kindle-calendar-v0.2 (Autodesk Fusion 360 design; units mm, degrees)
part number: 2026-08-25-10-04-39-781
part number: 2026-08-25-10-04-40-282
part number: 2026-08-25-10-04-41-157
part number: 2026-08-25-10-04-41-332
part number: 2026-08-25-10-04-41-515
part number: 2026-08-25-10-04-41-590
part number: 2026-08-25-10-04-41-668
Autodesk Fusion 360 part; units mm, degrees
sketch "Outer biomorphic silhouette" plane through (0, 0, 0) normal (0, 0, 1) x (1, 0, 0) in component "01 Asymmetric Front Shell"
  spline S0 degree 5 poles (-110, 58) (-109.8536, 58.1992) (-109.5513, 58.5949) (-109.0687, 59.1811) (-108.3683, 59.9478) (-107.4137, 60.8802) (-106.4012, 61.7844) (-105.3501, 62.6585) (-104.2698, 63.5023) (-103.1612, 64.3169) (-102.0207, 65.104) (-100.843, 65.8656) (-99.6254, 66.6035) (-98.369, 67.3186) (-97.0773, 68.0113) (-95.7548, 68.682) (-94.406, 69.3309) (-93.0336, 69.9586) (-91.6389, 70.5656) (-90.2223, 71.1528) (-88.7835, 71.7209) (-87.3225, 72.2707) (-85.8396, 72.8028) (-84.3357, 73.3177) (-82.8123, 73.8158) (-81.2704, 74.2975) (-79.7114, 74.7631) (-78.1363, 75.213) (-76.5457, 75.6475) (-74.9401, 76.0671) (-73.3198, 76.472) (-71.6854, 76.8628) (-70.0371, 77.2395) (-68.3753, 77.6027) (-66.7008, 77.9525) (-65.014, 78.2891) (-63.3154, 78.6129) (-61.6055, 78.9239) (-59.8849, 79.2225) (-58.154, 79.5088) (-56.413, 79.7831) (-54.6623, 80.0454) (-52.9022, 80.2961) (-51.1331, 80.5352) (-49.3552, 80.7629) (-47.569, 80.9795) (-45.7747, 81.1849) (-43.9727, 81.3794) (-42.1632, 81.5631) (-40.3466, 81.7361) (-38.5232, 81.8984) (-36.6932, 82.0503) (-34.8569, 82.1918) (-33.0145, 82.323) (-31.1664, 82.4441) (-29.3127, 82.555) (-27.4537, 82.6559) (-25.5896, 82.7469) (-23.7207, 82.828) (-21.8472, 82.8993) (-19.9693, 82.9608) (-18.0873, 83.0127) (-16.2014, 83.055) (-14.3119, 83.0877) (-12.4188, 83.1108) (-10.5225, 83.1245) (-8.6232, 83.1287) (-6.721, 83.1236) (-4.8162, 83.109) (-2.9089, 83.0852) (-0.9993, 83.052) (0.9123, 83.0096) (2.8257, 82.9579) (4.7408, 82.897) (6.6574, 82.8269) (8.5752, 82.7476) (10.4939, 82.659) (12.4135, 82.5612) (14.3337, 82.4542) (16.2544, 82.338) (18.1754, 82.2127) (20.0965, 82.0781) (22.0176, 81.9344) (23.9386, 81.7816) (25.8592, 81.6196) (27.7793, 81.4484) (29.6985, 81.268) (31.6165, 81.0782) (33.5331, 80.879) (35.4479, 80.6704) (37.3608, 80.4523) (39.2716, 80.2247) (41.1804, 79.9878) (43.0872, 79.7414) (44.9921, 79.4858) (46.8951, 79.221) (48.796, 78.9469) (50.6944, 78.6634) (52.5898, 78.3703) (54.4812, 78.0673) (56.3678, 77.754) (58.2491, 77.4301) (60.1245, 77.0957) (61.9943, 76.7506) (63.8591, 76.3953) (65.7201, 76.0303) (67.5784, 75.656) (69.4351, 75.273) (71.2902, 74.8814) (73.143, 74.4807) (74.991, 74.07) (76.8309, 73.6477) (78.659, 73.2124) (80.4724, 72.7628) (82.2696, 72.2982) (84.0519, 71.8192) (85.8237, 71.3278) (87.5923, 70.827) (89.3653, 70.3201) (91.1485, 69.8097) (92.944, 69.2966) (94.7479, 68.7792) (96.5478, 68.252) (98.3255, 67.7073) (100.0622, 67.1368) (101.7442, 66.5346) (103.3671, 65.899) (104.9414, 65.2342) (106.4984, 64.5538) (108.0806, 63.8762) (109.7297, 63.2194) (111.4739, 62.5956) (113.3164, 62.006) (115.2224, 61.4358) (117.1099, 60.8495) (118.8737, 60.2015) (120.4065, 59.4454) (121.6228, 58.5441) (122.4786, 57.4779) (122.9997, 56.2572) (123.2769, 54.9205) (123.4272, 53.5172) (123.5655, 52.0965) (123.7693, 50.6918) (124.054, 49.3103) (124.3966, 47.9433) (124.7539, 46.5733) (125.0817, 45.1826) (125.3572, 43.762) (125.5811, 42.3127) (125.7671, 40.8409) (125.9346, 39.3553) (126.101, 37.8636) (126.2728, 36.3692) (126.4483, 34.8719) (126.621, 33.3695) (126.7829, 31.8589) (126.9273, 30.3379) (127.0523, 28.8062) (127.1592, 27.2646) (127.2508, 25.7149) (127.3308, 24.159) (127.4019, 22.5985) (127.465, 21.034) (127.5196, 19.4659) (127.5644, 17.894) (127.5979, 16.3181) (127.619, 14.738) (127.6273, 13.154) (127.6229, 11.5666) (127.6064, 9.9763) (127.5784, 8.3839) (127.5393, 6.7898) (127.4893, 5.1945) (127.4283, 3.5985) (127.3559, 2.002) (127.2718, 0.4052) (127.1757, -1.1915) (127.0675, -2.788) (126.947, -4.3838) (126.8142, -5.9786) (126.6692, -7.572) (126.5119, -9.1635) (126.3422, -10.7526) (126.16, -12.339) (125.9651, -13.9221) (125.7573, -15.5016) (125.5363, -17.077) (125.302, -18.6481) (125.0543, -20.2147) (124.7929, -21.7765) (124.5177, -23.3334) (124.2285, -24.8846) (123.925, -26.4296) (123.607, -27.9673) (123.2741, -29.4968) (122.926, -31.0172) (122.5624, -32.5281) (122.1832, -34.0297) (121.7881, -35.5227) (121.377, -37.0074) (120.9497, -38.4841) (120.5056, -39.9519) (120.0444, -41.4085) (119.5652, -42.8504) (119.0673, -44.2743) (118.5502, -45.678) (118.0136, -47.0616) (117.4574, -48.4288) (116.882, -49.7855) (116.2877, -51.1365) (115.6741, -52.4832) (115.0403, -53.8207) (114.3843, -55.1352) (113.7035, -56.4096) (112.996, -57.6312) (112.2611, -58.797) (111.5002, -59.9229) (110.717, -61.0429) (109.915, -62.1908) (109.0958, -63.3842) (108.2575, -64.6092) (107.3916, -65.8006) (106.4871, -66.8662) (105.5344, -67.7206) (104.5298, -68.3118) (103.4799, -68.6609) (102.4017, -68.8585) (101.3139, -69.0113) (100.2312, -69.2048) (99.157, -69.4545) (98.087, -69.7325) (97.0134, -69.9954) (95.9293, -70.2157) (94.8311, -70.3967) (93.7186, -70.5537) (92.5947, -70.7053) (91.4659, -70.8577) (90.3388, -71.0076) (89.2161, -71.1477) (88.0919, -71.2722) (86.9489, -71.3805) (85.771, -71.4751) (84.5521, -71.5599) (83.3097, -71.6374) (82.084, -71.7082) (80.9096, -71.7718) (79.7971, -71.8272) (78.7032, -71.8739) (77.537, -71.9118) (76.1974, -71.9414) (74.6001, -71.9637) (72.715, -71.9795) (70.5721, -71.9899) (68.2401, -71.9961) (65.812, -71.9993) (63.389, -72.0003) (61.0632, -72.0003) (58.9037, -71.9998) (56.9362, -71.9993) (55.142, -71.9992) (53.4753, -71.9993) (51.8752, -71.9996) (50.2802, -72) (48.6412, -72.0003) (46.9367, -72.0004) (45.1685, -72.0004) (43.3535, -72.0003) (41.5165, -72.0001) (39.6833, -72) (37.8724, -71.9999) (36.0898, -71.9998) (34.3326, -71.9998) (32.5923, -71.9999) (30.8576, -72) (29.1182, -72) (27.3678, -72.0001) (25.6053, -72.0001) (23.8329, -72.0001) (22.0548, -72) (20.276, -72) (18.5004, -72) (16.7299, -72) (14.9644, -72) (13.2026, -72) (11.4423, -72) (9.6817, -72) (7.9191, -72) (6.1544, -72) (4.3877, -72) (2.62, -72) (0.8522, -72) (-0.915, -72) (-2.6811, -72) (-4.4465, -72) (-6.2115, -72) (-7.9767, -72) (-9.7427, -72) (-11.5095, -72) (-13.2767, -72) (-15.0438, -72.0001) (-16.8099, -72.0001) (-18.5744, -72) (-20.3372, -72) (-22.0988, -71.9999) (-23.8606, -71.9999) (-25.6242, -71.9998) (-27.391, -71.9999) (-29.1619, -71.9999) (-30.9365, -72.0001) (-32.7126, -72.0002) (-34.4867, -72.0003) (-36.2552, -72.0004) (-38.015, -72.0003) (-39.7654, -72.0001) (-41.5084, -71.9997) (-43.2504, -71.9994) (-45, -71.9992) (-46.7655, -71.9992) (-48.5525, -71.9995) (-50.3617, -72.0001) (-52.1857, -72.0009) (-54.0082, -72.0019) (-55.8082, -72.0025) (-57.5645, -72.0026) (-59.2593, -72.0015) (-60.8822, -71.9988) (-62.4358, -71.9938) (-63.9338, -71.986) (-65.3961, -71.9748) (-66.8432, -71.9595) (-68.2915, -71.9398) (-69.7476, -71.9154) (-71.2093, -71.886) (-72.6694, -71.8516) (-74.1192, -71.8122) (-75.5518, -71.768) (-76.9654, -71.7192) (-78.3613, -71.6659) (-79.743, -71.6083) (-81.1137, -71.5459) (-82.4753, -71.4782) (-83.8275, -71.4043) (-85.1688, -71.3233) (-86.4975, -71.2349) (-87.8119, -71.1397) (-89.1112, -71.0391) (-90.3952, -70.9349) (-91.6641, -70.8275) (-92.9185, -70.7157) (-94.1589, -70.5951) (-95.3857, -70.4612) (-96.5986, -70.3116) (-97.7964, -70.1486) (-98.9764, -69.9814) (-100.1362, -69.8199) (-101.2743, -69.6687) (-102.3923, -69.5197) (-103.4947, -69.3489) (-104.5859, -69.1268) (-105.6673, -68.8256) (-106.733, -68.43) (-107.7721, -67.9375) (-108.7723, -67.3527) (-109.7243, -66.6839) (-110.6256, -65.9382) (-111.4785, -65.122) (-112.2874, -64.241) (-113.0566, -63.3006) (-113.7878, -62.3059) (-114.4821, -61.2616) (-115.1394, -60.1723) (-115.7605, -59.0417) (-116.3468, -57.8734) (-116.9003, -56.6703) (-117.4232, -55.4349) (-117.9176, -54.1697) (-118.3848, -52.8767) (-118.8262, -51.5579) (-119.2426, -50.2152) (-119.6348, -48.8502) (-120.0038, -47.4645) (-120.3505, -46.0593) (-120.6757, -44.636) (-120.9805, -43.1957) (-121.2656, -41.7396) (-121.5317, -40.2685) (-121.7796, -38.7835) (-122.0098, -37.2855) (-122.2227, -35.7753) (-122.4188, -34.2537) (-122.5987, -32.7216) (-122.7628, -31.1795) (-122.9115, -29.6283) (-123.0452, -28.0686) (-123.1643, -26.501) (-123.2691, -24.9262) (-123.3601, -23.3447) (-123.4374, -21.7571) (-123.5013, -20.164) (-123.5522, -18.5659) (-123.5901, -16.9633) (-123.6155, -15.3568) (-123.6284, -13.7469) (-123.629, -12.1341) (-123.6176, -10.5188) (-123.5944, -8.9016) (-123.5595, -7.2829) (-123.513, -5.6633) (-123.4552, -4.0431) (-123.386, -2.4228) (-123.3057, -0.803) (-123.2143, 0.8159) (-123.1118, 2.4336) (-122.9983, 4.0494) (-122.874, 5.663) (-122.7388, 7.2738) (-122.593, 8.8813) (-122.4365, 10.4852) (-122.2695, 12.0848) (-122.0919, 13.6796) (-121.9038, 15.2692) (-121.705, 16.8531) (-121.4953, 18.4308) (-121.2746, 20.0019) (-121.0429, 21.5656) (-120.8002, 23.1215) (-120.5467, 24.6688) (-120.2827, 26.2069) (-120.0083, 27.7351) (-119.7235, 29.2526) (-119.4279, 30.7589) (-119.1205, 32.2534) (-118.8005, 33.7357) (-118.4671, 35.2052) (-118.12, 36.6609) (-117.7599, 38.1017) (-117.3881, 39.5263) (-117.0062, 40.9331) (-116.6149, 42.3206) (-116.2133, 43.6879) (-115.7983, 45.0346) (-115.3649, 46.3605) (-114.9088, 47.6654) (-114.4282, 48.948) (-113.9259, 50.2053) (-113.4109, 51.4327) (-112.8926, 52.6248) (-112.3754, 53.7773) (-111.8541, 54.8885) (-111.3076, 55.9605) (-110.8269, 56.7905) (-110.4297, 57.3999) (-110.1464, 57.8008) (-110, 58) knots 0 0 0 0 0 0 0.00222222 0.00444444 0.00666667 0.00888889 0.01111111 0.01333333 0.01555556 0.01777778 0.02 0.02222222 0.02444444 0.02666667 0.02888889 0.03111111 0.03333333 0.03555556 0.03777778 0.04 0.04222222 0.04444444 0.04666667 0.04888889 0.05111111 0.05333333 0.05555556 0.05777778 0.06 0.06222222 0.06444444 0.06666667 0.06888889 0.07111111 0.07333333 0.07555556 0.07777778 0.08 0.08222222 0.08444444 0.08666667 0.08888889 0.09111111 0.09333333 0.09555556 0.09777778 0.1 0.10222222 0.10444444 0.10666667 0.10888889 0.11111111 0.11333333 0.11555556 0.11777778 0.12 0.12222222 0.12444444 0.12666667 0.12888889 0.13111111 0.13333333 0.13555556 0.13777778 0.14 0.14222222 0.14444444 0.14666667 0.14888889 0.15111111 0.15333333 0.15555556 0.15777778 0.16 0.16222222 0.16444444 0.16666667 0.16888889 0.17111111 0.17333333 0.17555556 0.17777778 0.18 0.18222222 0.18444444 0.18666667 0.18888889 0.19111111 0.19333333 0.19555556 0.19777778 0.2 0.20222222 0.20444444 0.20666667 0.20888889 0.21111111 0.21333333 0.21555556 0.21777778 0.22 0.22222222 0.22444444 0.22666667 0.22888889 0.23111111 0.23333333 0.23555556 0.23777778 0.24 0.24222222 0.24444444 0.24666667 0.24888889 0.25111111 0.25333333 0.25555556 0.25777778 0.26 0.26222222 0.26444444 0.26666667 0.26888889 0.27111111 0.27333333 0.27555556 0.27777778 0.28 0.28222222 0.28444444 0.28666667 0.28888889 0.29111111 0.29333333 0.29555556 0.29777778 0.3 0.30222222 0.30444444 0.30666667 0.30888889 0.31111111 0.31333333 0.31555556 0.31777778 0.32 0.32222222 0.32444444 0.32666667 0.32888889 0.33111111 0.33333333 0.33555556 0.33777778 0.34 0.34222222 0.34444444 0.34666667 0.34888889 0.35111111 0.35333333 0.35555556 0.35777778 0.36 0.36222222 0.36444444 0.36666667 0.36888889 0.37111111 0.37333333 0.37555556 0.37777778 0.38 0.38222222 0.38444444 0.38666667 0.38888889 0.39111111 0.39333333 0.39555556 0.39777778 0.4 0.40222222 0.40444444 0.40666667 0.40888889 0.41111111 0.41333333 0.41555556 0.41777778 0.42 0.42222222 0.42444444 0.42666667 0.42888889 0.43111111 0.43333333 0.43555556 0.43777778 0.44 0.44222222 0.44444444 0.44666667 0.44888889 0.45111111 0.45333333 0.45555556 0.45777778 0.46 0.46222222 0.46444444 0.46666667 0.46888889 0.47111111 0.47333333 0.47555556 0.47777778 0.48 0.48222222 0.48444444 0.48666667 0.48888889 0.49111111 0.49333333 0.49555556 0.49777778 0.5 0.50222222 0.50444444 0.50666667 0.50888889 0.51111111 0.51333333 0.51555556 0.51777778 0.52 0.52222222 0.52444444 0.52666667 0.52888889 0.53111111 0.53333333 0.53555556 0.53777778 0.54 0.54222222 0.54444444 0.54666667 0.54888889 0.55111111 0.55333333 0.55555556 0.55777778 0.56 0.56222222 0.56444444 0.56666667 0.56888889 0.57111111 0.57333333 0.57555556 0.57777778 0.58 0.58222222 0.58444444 0.58666667 0.58888889 0.59111111 0.59333333 0.59555556 0.59777778 0.6 0.60222222 0.60444444 0.60666667 0.60888889 0.61111111 0.61333333 0.61555556 0.61777778 0.62 0.62222222 0.62444444 0.62666667 0.62888889 0.63111111 0.63333333 0.63555556 0.63777778 0.64 0.64222222 0.64444444 0.64666667 0.64888889 0.65111111 0.65333333 0.65555556 0.65777778 0.66 0.66222222 0.66444444 0.66666667 0.66888889 0.67111111 0.67333333 0.67555556 0.67777778 0.68 0.68222222 0.68444444 0.68666667 0.68888889 0.69111111 0.69333333 0.69555556 0.69777778 0.7 0.70222222 0.70444444 0.70666667 0.70888889 0.71111111 0.71333333 0.71555556 0.71777778 0.72 0.72222222 0.72444444 0.72666667 0.72888889 0.73111111 0.73333333 0.73555556 0.73777778 0.74 0.74222222 0.74444444 0.74666667 0.74888889 0.75111111 0.75333333 0.75555556 0.75777778 0.76 0.76222222 0.76444444 0.76666667 0.76888889 0.77111111 0.77333333 0.77555556 0.77777778 0.78 0.78222222 0.78444444 0.78666667 0.78888889 0.79111111 0.79333333 0.79555556 0.79777778 0.8 0.80222222 0.80444444 0.80666667 0.80888889 0.81111111 0.81333333 0.81555556 0.81777778 0.82 0.82222222 0.82444444 0.82666667 0.82888889 0.83111111 0.83333333 0.83555556 0.83777778 0.84 0.84222222 0.84444444 0.84666667 0.84888889 0.85111111 0.85333333 0.85555556 0.85777778 0.86 0.86222222 0.86444444 0.86666667 0.86888889 0.87111111 0.87333333 0.87555556 0.87777778 0.88 0.88222222 0.88444444 0.88666667 0.88888889 0.89111111 0.89333333 0.89555556 0.89777778 0.9 0.90222222 0.90444444 0.90666667 0.90888889 0.91111111 0.91333333 0.91555556 0.91777778 0.92 0.92222222 0.92444444 0.92666667 0.92888889 0.93111111 0.93333333 0.93555556 0.93777778 0.94 0.94222222 0.94444444 0.94666667 0.94888889 0.95111111 0.95333333 0.95555556 0.95777778 0.96 0.96222222 0.96444444 0.96666667 0.96888889 0.97111111 0.97333333 0.97555556 0.97777778 0.98 0.98222222 0.98444444 0.98666667 0.98888889 0.99111111 0.99333333 0.99555556 0.99777778 1 1 1 1 1 1
  point P0 (-106.1798, 61.9581)
  point P1 (-101.272, 65.5816)
  point P2 (-95.3555, 68.8691)
  point P3 (-88.5093, 71.8194)
  point P4 (-80.8124, 74.4312)
  point P5 (-72.3438, 76.7031)
  point P6 (-63.1824, 78.6339)
  point P7 (-53.4074, 80.2222)
  point P8 (-43.0977, 81.4668)
  point P9 (-32.3322, 82.3663)
  point P10 (-21.19, 82.9195)
  point P11 (-9.75, 83.125)
  point P12 (1.9087, 82.9816)
  point P13 (13.7072, 82.4878)
  point P14 (25.5664, 81.6426)
  point P15 (37.4074, 80.4444)
  point P16 (49.1512, 78.8921)
  point P17 (60.7188, 76.9844)
  point P18 (72.0311, 74.7198)
  point P19 (83.0093, 72.0972)
  point P20 (93.5742, 69.1152)
  point P21 (103.647, 65.7726)
  point P22 (113.1486, 62.0679)
  point P23 (122, 58)
  point P24 (123.5537, 52.3292)
  point P25 (124.8738, 46.0412)
  point P26 (125.9491, 39.2222)
  point P27 (126.7682, 31.9588)
  point P28 (127.3198, 24.3374)
  point P29 (127.5926, 16.4444)
  point P30 (127.5753, 8.3663)
  point P31 (127.2565, 0.1893)
  point P32 (126.625, -8)
  point P33 (125.6694, -16.1152)
  point P34 (124.3784, -24.07)
  point P35 (122.7407, -31.7778)
  point P36 (120.745, -39.1523)
  point P37 (118.38, -46.107)
  point P38 (115.6343, -52.5556)
  point P39 (112.4966, -58.4115)
  point P40 (108.9556, -63.5885)
  point P41 (105, -68)
  point P42 (101.2402, -69.0332)
  point P43 (97.4219, -69.8906)
  point P44 (93.4863, -70.584)
  point P45 (89.375, -71.125)
  point P46 (85.0293, -71.5254)
  point P47 (80.3906, -71.7969)
  point P48 (75.4004, -71.9512)
  point P49 (60, -72)
  point P50 (50, -72)
  point P51 (40, -72)
  point P52 (30, -72)
  point P53 (20, -72)
  point P54 (10, -72)
  point P55 (0, -72)
  point P56 (-10, -72)
  point P57 (-20, -72)
  point P58 (-30, -72)
  point P59 (-40, -72)
  point P60 (-50, -72)
  point P61 (-60, -72)
  point P62 (-67.2656, -71.9531)
  point P63 (-74.0625, -71.8125)
  point P64 (-80.3906, -71.5781)
  point P65 (-86.25, -71.25)
  point P66 (-91.6406, -70.8281)
  point P67 (-96.5625, -70.3125)
  point P68 (-101.0156, -69.7031)
  point P69 (-105, -69)
  point P70 (-108.8054, -67.3026)
  point P71 (-112.133, -64.391)
  point P72 (-115.0001, -60.3859)
  point P73 (-117.424, -55.408)
  point P74 (-119.4219, -49.5781)
  point P75 (-121.011, -43.017)
  point P76 (-122.2086, -35.8454)
  point P77 (-123.032, -28.184)
  point P78 (-123.4984, -20.1536)
  point P79 (-123.625, -11.875)
  point P80 (-123.4291, -3.4689)
  point P81 (-122.928, 4.944)
  point P82 (-122.1389, 13.2429)
  point P83 (-121.079, 21.307)
  point P84 (-119.7656, 29.0156)
  point P85 (-118.216, 36.248)
  point P86 (-116.4474, 42.8834)
  point P87 (-114.477, 48.801)
  point P88 (-112.3221, 53.8801)
extrude "Asymmetric shell" add sketch "Outer biomorphic silhouette" along normal blind 15 makes body 1 in component "01 Asymmetric Front Shell"
sketch "Visible e-ink aperture" plane through (0, 0, 0) normal (0, 0, 1) x (1, 0, 0) in component "01 Asymmetric Front Shell"
  line L0 (-44.85, -41.65) -> (72.85, -41.65)
  line L1 (74.85, -39.65) -> (74.85, 47.65)
  line L2 (72.85, 49.65) -> (-44.85, 49.65)
  line L3 (-46.85, 47.65) -> (-46.85, -39.65)
  arc A0 (72.85, -41.65) -> (74.85, -39.65) centre (72.85, -39.65) ccw
  arc A1 (74.85, 47.65) -> (72.85, 49.65) centre (72.85, 47.65) ccw
  arc A2 (-44.85, 49.65) -> (-46.85, 47.65) centre (-44.85, 47.65) ccw
  arc A3 (-46.85, -39.65) -> (-44.85, -41.65) centre (-44.85, -39.65) ccw
  constraint tangent L0 A0
  constraint tangent L1 A0
  constraint tangent L1 A1
  constraint tangent L2 A1
  constraint tangent L2 A2
  constraint tangent L3 A2
  constraint tangent L3 A3
  constraint tangent L0 A3
extrude "Cut screen aperture" cut sketch "Visible e-ink aperture" along normal blind 15 bodies 1 in component "01 Asymmetric Front Shell"
sketch "Asymmetric negative-space opening" plane through (0, 0, 0) normal (0, 0, 1) x (1, 0, 0) in component "01 Asymmetric Front Shell"
  spline S0 degree 5 poles (-80, -1) (-80, -0.8461) (-80.0011, -0.5384) (-80.0062, -0.0768) (-80.0197, 0.5385) (-80.0479, 1.3068) (-80.0873, 2.0741) (-80.138, 2.84) (-80.2, 3.604) (-80.2734, 4.366) (-80.3581, 5.1253) (-80.4541, 5.8818) (-80.5615, 6.6351) (-80.6803, 7.3846) (-80.8106, 8.1302) (-80.9523, 8.8713) (-81.1056, 9.6075) (-81.2704, 10.3385) (-81.4468, 11.0638) (-81.6349, 11.783) (-81.8346, 12.4956) (-82.0462, 13.2011) (-82.2695, 13.8992) (-82.5047, 14.5893) (-82.7518, 15.2708) (-83.0109, 15.9434) (-83.2821, 16.6063) (-83.5654, 17.2591) (-83.8608, 17.9012) (-84.1686, 18.5318) (-84.4886, 19.1505) (-84.8211, 19.7564) (-85.166, 20.3489) (-85.5234, 20.9272) (-85.8933, 21.4906) (-86.2759, 22.0381) (-86.6711, 22.569) (-87.0789, 23.0822) (-87.4993, 23.5769) (-87.9322, 24.0519) (-88.3777, 24.5062) (-88.8356, 24.9387) (-89.3056, 25.3482) (-89.7876, 25.7334) (-90.2813, 26.093) (-90.7862, 26.4258) (-91.3019, 26.7305) (-91.8278, 27.0056) (-92.3631, 27.2498) (-92.907, 27.462) (-93.4584, 27.6408) (-94.0163, 27.7854) (-94.5792, 27.8946) (-95.146, 27.9678) (-95.7151, 28.0046) (-96.2849, 28.0046) (-96.854, 27.9678) (-97.4208, 27.8946) (-97.9837, 27.7854) (-98.5416, 27.6408) (-99.093, 27.462) (-99.6369, 27.2498) (-100.1722, 27.0056) (-100.6981, 26.7305) (-101.2138, 26.4258) (-101.7187, 26.093) (-102.2124, 25.7334) (-102.6944, 25.3482) (-103.1644, 24.9387) (-103.6223, 24.5062) (-104.0678, 24.0519) (-104.5007, 23.5769) (-104.9211, 23.0822) (-105.3289, 22.569) (-105.7241, 22.0381) (-106.1067, 21.4906) (-106.4766, 20.9272) (-106.834, 20.3489) (-107.1789, 19.7564) (-107.5114, 19.1505) (-107.8314, 18.5318) (-108.1392, 17.9012) (-108.4346, 17.2591) (-108.7179, 16.6063) (-108.9891, 15.9434) (-109.2482, 15.2708) (-109.4953, 14.5893) (-109.7305, 13.8992) (-109.9538, 13.2011) (-110.1654, 12.4956) (-110.3651, 11.783) (-110.5532, 11.0638) (-110.7296, 10.3385) (-110.8944, 9.6075) (-111.0477, 8.8713) (-111.1894, 8.1302) (-111.3197, 7.3846) (-111.4385, 6.6351) (-111.5459, 5.8818) (-111.6419, 5.1253) (-111.7266, 4.366) (-111.8, 3.604) (-111.862, 2.84) (-111.9127, 2.0741) (-111.9521, 1.3068) (-111.9803, 0.5385) (-111.9972, -0.2306) (-112.0028, -1) (-111.9972, -1.7694) (-111.9803, -2.5385) (-111.9521, -3.3068) (-111.9127, -4.0741) (-111.862, -4.84) (-111.8, -5.604) (-111.7266, -6.366) (-111.6419, -7.1253) (-111.5459, -7.8818) (-111.4385, -8.6351) (-111.3197, -9.3846) (-111.1894, -10.1302) (-111.0477, -10.8713) (-110.8944, -11.6075) (-110.7296, -12.3385) (-110.5532, -13.0638) (-110.3651, -13.783) (-110.1654, -14.4956) (-109.9538, -15.2011) (-109.7305, -15.8992) (-109.4953, -16.5893) (-109.2482, -17.2708) (-108.9891, -17.9434) (-108.7179, -18.6063) (-108.4346, -19.2591) (-108.1392, -19.9012) (-107.8314, -20.5318) (-107.5114, -21.1505) (-107.1789, -21.7564) (-106.834, -22.3489) (-106.4766, -22.9272) (-106.1067, -23.4906) (-105.7241, -24.0381) (-105.3289, -24.569) (-104.9211, -25.0822) (-104.5007, -25.5769) (-104.0678, -26.0519) (-103.6223, -26.5062) (-103.1644, -26.9387) (-102.6944, -27.3482) (-102.2124, -27.7334) (-101.7187, -28.093) (-101.2138, -28.4258) (-100.6981, -28.7305) (-100.1722, -29.0056) (-99.6369, -29.2498) (-99.093, -29.462) (-98.5416, -29.6408) (-97.9837, -29.7854) (-97.4208, -29.8946) (-96.854, -29.9678) (-96.2849, -30.0046) (-95.7151, -30.0046) (-95.146, -29.9678) (-94.5792, -29.8946) (-94.0163, -29.7854) (-93.4584, -29.6408) (-92.907, -29.462) (-92.3631, -29.2498) (-91.8278, -29.0056) (-91.3019, -28.7305) (-90.7862, -28.4258) (-90.2813, -28.093) (-89.7876, -27.7334) (-89.3056, -27.3482) (-88.8356, -26.9387) (-88.3777, -26.5062) (-87.9322, -26.0519) (-87.4993, -25.5769) (-87.0789, -25.0822) (-86.6711, -24.569) (-86.2759, -24.0381) (-85.8933, -23.4906) (-85.5234, -22.9272) (-85.166, -22.3489) (-84.8211, -21.7564) (-84.4886, -21.1505) (-84.1686, -20.5318) (-83.8608, -19.9012) (-83.5654, -19.2591) (-83.2821, -18.6063) (-83.0109, -17.9434) (-82.7518, -17.2708) (-82.5047, -16.5893) (-82.2695, -15.8992) (-82.0462, -15.2011) (-81.8346, -14.4956) (-81.6349, -13.783) (-81.4468, -13.0638) (-81.2704, -12.3385) (-81.1056, -11.6075) (-80.9523, -10.8713) (-80.8106, -10.1302) (-80.6803, -9.3846) (-80.5615, -8.6351) (-80.4541, -7.8818) (-80.3581, -7.1253) (-80.2734, -6.366) (-80.2, -5.604) (-80.138, -4.84) (-80.0873, -4.0741) (-80.0479, -3.3068) (-80.0197, -2.5385) (-80.0062, -1.9232) (-80.0011, -1.4616) (-80, -1.1539) (-80, -1) knots 0 0 0 0 0 0 0.0047619 0.00952381 0.01428571 0.01904762 0.02380952 0.02857143 0.03333333 0.03809524 0.04285714 0.04761905 0.05238095 0.05714286 0.06190476 0.06666667 0.07142857 0.07619048 0.08095238 0.08571429 0.09047619 0.0952381 0.1 0.1047619 0.10952381 0.11428571 0.11904762 0.12380952 0.12857143 0.13333333 0.13809524 0.14285714 0.14761905 0.15238095 0.15714286 0.16190476 0.16666667 0.17142857 0.17619048 0.18095238 0.18571429 0.19047619 0.1952381 0.2 0.2047619 0.20952381 0.21428571 0.21904762 0.22380952 0.22857143 0.23333333 0.23809524 0.24285714 0.24761905 0.25238095 0.25714286 0.26190476 0.26666667 0.27142857 0.27619048 0.28095238 0.28571429 0.29047619 0.2952381 0.3 0.3047619 0.30952381 0.31428571 0.31904762 0.32380952 0.32857143 0.33333333 0.33809524 0.34285714 0.34761905 0.35238095 0.35714286 0.36190476 0.36666667 0.37142857 0.37619048 0.38095238 0.38571429 0.39047619 0.3952381 0.4 0.4047619 0.40952381 0.41428571 0.41904762 0.42380952 0.42857143 0.43333333 0.43809524 0.44285714 0.44761905 0.45238095 0.45714286 0.46190476 0.46666667 0.47142857 0.47619048 0.48095238 0.48571429 0.49047619 0.4952381 0.5 0.5047619 0.50952381 0.51428571 0.51904762 0.52380952 0.52857143 0.53333333 0.53809524 0.54285714 0.54761905 0.55238095 0.55714286 0.56190476 0.56666667 0.57142857 0.57619048 0.58095238 0.58571429 0.59047619 0.5952381 0.6 0.6047619 0.60952381 0.61428571 0.61904762 0.62380952 0.62857143 0.63333333 0.63809524 0.64285714 0.64761905 0.65238095 0.65714286 0.66190476 0.66666667 0.67142857 0.67619048 0.68095238 0.68571429 0.69047619 0.6952381 0.7 0.7047619 0.70952381 0.71428571 0.71904762 0.72380952 0.72857143 0.73333333 0.73809524 0.74285714 0.74761905 0.75238095 0.75714286 0.76190476 0.76666667 0.77142857 0.77619048 0.78095238 0.78571429 0.79047619 0.7952381 0.8 0.8047619 0.80952381 0.81428571 0.81904762 0.82380952 0.82857143 0.83333333 0.83809524 0.84285714 0.84761905 0.85238095 0.85714286 0.86190476 0.86666667 0.87142857 0.87619048 0.88095238 0.88571429 0.89047619 0.8952381 0.9 0.9047619 0.90952381 0.91428571 0.91904762 0.92380952 0.92857143 0.93333333 0.93809524 0.94285714 0.94761905 0.95238095 0.95714286 0.96190476 0.96666667 0.97142857 0.97619048 0.98095238 0.98571429 0.99047619 0.9952381 1 1 1 1 1 1
  point P0 (-80.1787, 3.3222)
  point P1 (-80.7108, 7.5479)
  point P2 (-81.5845, 11.5826)
  point P3 (-82.7802, 15.3363)
  point P4 (-84.2712, 18.725)
  point P5 (-86.0242, 21.6731)
  point P6 (-88, 24.1147)
  point P7 (-90.1545, 25.9953)
  point P8 (-92.4397, 27.2729)
  point P9 (-94.8043, 27.9189)
  point P10 (-97.1957, 27.9189)
  point P11 (-99.5603, 27.2729)
  point P12 (-101.8455, 25.9953)
  point P13 (-104, 24.1147)
  point P14 (-105.9758, 21.6731)
  point P15 (-107.7288, 18.725)
  point P16 (-109.2198, 15.3363)
  point P17 (-110.4155, 11.5826)
  point P18 (-111.2892, 7.5479)
  point P19 (-111.8213, 3.3222)
  point P20 (-112, -1)
  point P21 (-111.8213, -5.3222)
  point P22 (-111.2892, -9.5479)
  point P23 (-110.4155, -13.5826)
  point P24 (-109.2198, -17.3363)
  point P25 (-107.7288, -20.725)
  point P26 (-105.9758, -23.6731)
  point P27 (-104, -26.1147)
  point P28 (-101.8455, -27.9953)
  point P29 (-99.5603, -29.2729)
  point P30 (-97.1957, -29.9189)
  point P31 (-94.8043, -29.9189)
  point P32 (-92.4397, -29.2729)
  point P33 (-90.1545, -27.9953)
  point P34 (-88, -26.1147)
  point P35 (-86.0242, -23.6731)
  point P36 (-84.2712, -20.725)
  point P37 (-82.7802, -17.3363)
  point P38 (-81.5845, -13.5826)
  point P39 (-80.7108, -9.5479)
  point P40 (-80.1787, -5.3222)
extrude "Cut sculptural opening" cut sketch "Asymmetric negative-space opening" along normal blind 15 bodies 1 in component "01 Asymmetric Front Shell"
ref_plane "WorkPlane1" through (0, 0, 3.2) normal (0, 0, 1) x (1, 0, 0) in component "01 Asymmetric Front Shell"
sketch "Rear-loading Kindle pocket" plane through (0, 0, 3.2) normal (0, 0, 1) x (1, 0, 0) in component "01 Asymmetric Front Shell"
  line L0 (-61.6, -54.6) -> (94.6, -54.6)
  line L1 (100.1, -49.1) -> (100.1, 55.1)
  line L2 (94.6, 60.6) -> (-61.6, 60.6)
  line L3 (-67.1, 55.1) -> (-67.1, -49.1)
  arc A0 (94.6, -54.6) -> (100.1, -49.1) centre (94.6, -49.1) ccw
  arc A1 (100.1, 55.1) -> (94.6, 60.6) centre (94.6, 55.1) ccw
  arc A2 (-61.6, 60.6) -> (-67.1, 55.1) centre (-61.6, 55.1) ccw
  arc A3 (-67.1, -49.1) -> (-61.6, -54.6) centre (-61.6, -49.1) ccw
  constraint tangent L0 A0
  constraint tangent L1 A0
  constraint tangent L1 A1
  constraint tangent L2 A1
  constraint tangent L2 A2
  constraint tangent L3 A2
  constraint tangent L3 A3
  constraint tangent L0 A3
extrude "Cut Kindle pocket" cut sketch "Rear-loading Kindle pocket" along normal blind 11.8 bodies 1 in component "01 Asymmetric Front Shell"
sketch "USB plug bay" plane through (0, 0, 3.2) normal (0, 0, 1) x (1, 0, 0) in component "01 Asymmetric Front Shell"
  line L0 (101.1, -7) -> (113.1, -7)
  line L1 (116.1, -4) -> (116.1, 16)
  line L2 (113.1, 19) -> (101.1, 19)
  line L3 (98.1, 16) -> (98.1, -4)
  arc A0 (113.1, -7) -> (116.1, -4) centre (113.1, -4) ccw
  arc A1 (116.1, 16) -> (113.1, 19) centre (113.1, 16) ccw
  arc A2 (101.1, 19) -> (98.1, 16) centre (101.1, 16) ccw
  arc A3 (98.1, -4) -> (101.1, -7) centre (101.1, -4) ccw
  constraint tangent L0 A0
  constraint tangent L1 A0
  constraint tangent L1 A1
  constraint tangent L2 A1
  constraint tangent L2 A2
  constraint tangent L3 A2
  constraint tangent L3 A3
  constraint tangent L0 A3
extrude "Cut USB plug bay" cut sketch "USB plug bay" along normal blind 11.8 bodies 1 in component "01 Asymmetric Front Shell"
sketch "USB cable channel" plane through (0, 0, 3.2) normal (0, 0, 1) x (1, 0, 0) in component "01 Asymmetric Front Shell"
  line L0 (105.1, -81) -> (109.1, -81)
  line L1 (112.1, -78) -> (112.1, -6)
  line L2 (109.1, -3) -> (105.1, -3)
  line L3 (102.1, -6) -> (102.1, -78)
  arc A0 (109.1, -81) -> (112.1, -78) centre (109.1, -78) ccw
  arc A1 (112.1, -6) -> (109.1, -3) centre (109.1, -6) ccw
  arc A2 (105.1, -3) -> (102.1, -6) centre (105.1, -6) ccw
  arc A3 (102.1, -78) -> (105.1, -81) centre (105.1, -78) ccw
  constraint tangent L0 A0
  constraint tangent L1 A0
  constraint tangent L1 A1
  constraint tangent L2 A1
  constraint tangent L2 A2
  constraint tangent L3 A2
  constraint tangent L3 A3
  constraint tangent L0 A3
extrude "Cut cable channel" cut sketch "USB cable channel" along normal blind 11.8 bodies 1 in component "01 Asymmetric Front Shell"
ref_plane "WorkPlane2" through (0, 0, 15.25) normal (0, 0, 1) x (1, 0, 0) in component "01 Asymmetric Front Shell"
sketch "Cover screw pilots" plane through (0, 0, 15.25) normal (0, 0, 1) x (1, 0, 0) in component "01 Asymmetric Front Shell"
  circle A0 centre (16.5, 64.8) radius 1.1
  circle A1 centre (16.5, -58.8) radius 1.1
  circle A2 centre (-71.3, 3) radius 1.1
  circle A3 centre (104.3, 34) radius 1.1
extrude "Cut cover screw pilots" cut sketch "Cover screw pilots" against normal blind 8 bodies 1 in component "01 Asymmetric Front Shell"
sketch "Hood pin holes" plane through (0, 0, 0) normal (0, 0, 1) x (1, 0, 0) in component "01 Asymmetric Front Shell"
  circle A0 centre (-50, 75) radius 2.2
  circle A1 centre (80, 72) radius 2.2
extrude "Cut hood pin holes" cut sketch "Hood pin holes" along normal blind 6.5 bodies 1 in component "01 Asymmetric Front Shell"
ref_plane "WorkPlane1" through (0, 0, 15.25) normal (0, 0, 1) x (1, 0, 0) in component "02 Rear Cover"
sketch "Rear cover outline" plane through (0, 0, 15.25) normal (0, 0, 1) x (1, 0, 0) in component "02 Rear Cover"
  line L0 (-68.5, -63) -> (101.5, -63)
  line L1 (108.5, -56) -> (108.5, 62)
  line L2 (101.5, 69) -> (-68.5, 69)
  line L3 (-75.5, 62) -> (-75.5, -56)
  arc A0 (101.5, -63) -> (108.5, -56) centre (101.5, -56) ccw
  arc A1 (108.5, 62) -> (101.5, 69) centre (101.5, 62) ccw
  arc A2 (-68.5, 69) -> (-75.5, 62) centre (-68.5, 62) ccw
  arc A3 (-75.5, -56) -> (-68.5, -63) centre (-68.5, -56) ccw
  constraint tangent L0 A0
  constraint tangent L1 A0
  constraint tangent L1 A1
  constraint tangent L2 A1
  constraint tangent L2 A2
  constraint tangent L3 A2
  constraint tangent L3 A3
  constraint tangent L0 A3
extrude "Rear cover" add sketch "Rear cover outline" along normal blind 2.8 separate body makes body 2 in component "02 Rear Cover"
sketch "Kindle press bosses" plane through (0, 0, 15.25) normal (0, 0, 1) x (1, 0, 0) in component "02 Rear Cover"
  circle A0 centre (-48.5, -37) radius 4
  circle A1 centre (-48.5, 43) radius 4
  circle A2 centre (81.5, -37) radius 4
  circle A3 centre (81.5, 43) radius 4
extrude "Press bosses" add sketch "Kindle press bosses" against normal blind 2.85 bodies 2 in component "02 Rear Cover"
sketch "Cover screw holes" plane through (0, 0, 15.25) normal (0, 0, 1) x (1, 0, 0) in component "02 Rear Cover"
  circle A0 centre (16.5, 64.8) radius 1.4
  circle A1 centre (16.5, -58.8) radius 1.4
  circle A2 centre (-71.3, 3) radius 1.4
  circle A3 centre (104.3, 34) radius 1.4
extrude "Cut screw holes" cut sketch "Cover screw holes" along normal blind 2.8 bodies 2 in component "02 Rear Cover"
sketch "USB notch" plane through (0, 0, 15.25) normal (0, 0, 1) x (1, 0, 0) in component "02 Rear Cover"
  line L0 (103.5, -3) -> (113.5, -3)
  line L1 (116.5, 0) -> (116.5, 12)
  line L2 (113.5, 15) -> (103.5, 15)
  line L3 (100.5, 12) -> (100.5, 0)
  arc A0 (113.5, -3) -> (116.5, 0) centre (113.5, 0) ccw
  arc A1 (116.5, 12) -> (113.5, 15) centre (113.5, 12) ccw
  arc A2 (103.5, 15) -> (100.5, 12) centre (103.5, 12) ccw
  arc A3 (100.5, 0) -> (103.5, -3) centre (103.5, 0) ccw
  constraint tangent L0 A0
  constraint tangent L1 A0
  constraint tangent L1 A1
  constraint tangent L2 A1
  constraint tangent L2 A2
  constraint tangent L3 A2
  constraint tangent L3 A3
  constraint tangent L0 A3
extrude "Cut USB notch" cut sketch "USB notch" along normal blind 2.8 bodies 2 in component "02 Rear Cover"
ref_plane "WorkPlane1" through (0, 0, -14) normal (0, 0, 1) x (1, 0, 0) in component "03 Front-Light Hood"
sketch "Cantilevered light hood" plane through (0, 0, -14) normal (0, 0, 1) x (1, 0, 0) in component "03 Front-Light Hood"
  spline S0 degree 5 poles (-111, 57) (-111.0367, 57.1832) (-110.9965, 57.5522) (-110.6065, 58.1104) (-109.5238, 58.8542) (-107.6226, 59.7665) (-105.5879, 60.652) (-103.7416, 61.5069) (-102.181, 62.331) (-100.8404, 63.1266) (-99.5743, 63.8975) (-98.2269, 64.647) (-96.7227, 65.3772) (-95.0712, 66.0885) (-93.3249, 66.7804) (-91.5535, 67.4521) (-89.8081, 68.1032) (-88.0994, 68.7339) (-86.414, 69.3449) (-84.7258, 69.9372) (-83.0082, 70.5118) (-81.2482, 71.0691) (-79.4473, 71.6096) (-77.6147, 72.1334) (-75.7632, 72.6406) (-73.9036, 73.1313) (-72.0403, 73.6058) (-70.1725, 74.0643) (-68.2965, 74.5073) (-66.4075, 74.9349) (-64.5022, 75.3476) (-62.5799, 75.7455) (-60.6418, 76.1289) (-58.6903, 76.4979) (-56.7279, 76.8527) (-54.7567, 77.1935) (-52.7774, 77.5203) (-50.7902, 77.8333) (-48.7946, 78.1328) (-46.7899, 78.4189) (-44.7759, 78.6917) (-42.7527, 78.9513) (-40.7208, 79.1979) (-38.6808, 79.4316) (-36.6334, 79.6525) (-34.5793, 79.8607) (-32.5189, 80.0562) (-30.4523, 80.2392) (-28.3799, 80.4098) (-26.3017, 80.568) (-24.2178, 80.7139) (-22.1284, 80.8476) (-20.0339, 80.9691) (-17.9344, 81.0785) (-15.8305, 81.1758) (-13.7222, 81.2612) (-11.6101, 81.3346) (-9.4943, 81.396) (-7.3751, 81.4456) (-5.2527, 81.4834) (-3.1273, 81.5093) (-0.9991, 81.5235) (1.1316, 81.5259) (3.2647, 81.5165) (5.3999, 81.4953) (7.5371, 81.4624) (9.6758, 81.4177) (11.816, 81.3613) (13.9571, 81.2932) (16.0991, 81.2134) (18.2415, 81.1219) (20.3842, 81.0187) (22.527, 80.9038) (24.67, 80.777) (26.8131, 80.6383) (28.9561, 80.4877) (31.0988, 80.3251) (33.2408, 80.1505) (35.3816, 79.964) (37.5205, 79.7657) (39.6569, 79.5556) (41.7905, 79.3338) (43.9213, 79.1) (46.0497, 78.854) (48.1764, 78.5956) (50.3021, 78.3244) (52.427, 78.0403) (54.5507, 77.7431) (56.6717, 77.4333) (58.7877, 77.1112) (60.8964, 76.7774) (62.9958, 76.4322) (65.0856, 76.0756) (67.1674, 75.707) (69.2454, 75.325) (71.3243, 74.9282) (73.4082, 74.5153) (75.4983, 74.0857) (77.5918, 73.64) (79.6795, 73.1807) (81.7493, 72.7107) (83.79, 72.233) (85.7957, 71.749) (87.7687, 71.2577) (89.7257, 70.7545) (91.6935, 70.2317) (93.6985, 69.6817) (95.7572, 69.0997) (97.8679, 68.486) (99.9985, 67.8492) (102.0875, 67.2058) (104.0707, 66.5733) (105.9021, 65.9641) (107.5759, 65.3795) (109.1528, 64.8024) (110.7689, 64.1951) (112.576, 63.5152) (114.6913, 62.7303) (117.1451, 61.8314) (119.8242, 60.8494) (122.4342, 59.8648) (124.6017, 58.9802) (125.9629, 58.2961) (126.2541, 57.8864) (125.4098, 57.771) (123.6321, 57.8977) (121.2716, 58.1738) (118.724, 58.4939) (116.3314, 58.7669) (114.256, 58.9493) (112.4807, 59.0459) (110.8897, 59.0876) (109.3258, 59.1166) (107.6567, 59.1682) (105.8391, 59.2541) (103.894, 59.3689) (101.8785, 59.4973) (99.8599, 59.6214) (97.886, 59.7287) (95.9664, 59.8165) (94.0878, 59.8887) (92.2242, 59.9521) (90.3475, 60.0143) (88.4412, 60.0798) (86.5037, 60.1491) (84.5424, 60.2204) (82.569, 60.2905) (80.5954, 60.3563) (78.628, 60.4162) (76.6671, 60.4702) (74.7094, 60.5191) (72.7501, 60.5644) (70.7845, 60.6074) (68.8102, 60.6487) (66.8276, 60.6883) (64.8383, 60.7258) (62.8446, 60.7606) (60.8489, 60.7922) (58.8521, 60.8203) (56.8544, 60.8449) (54.8553, 60.8663) (52.8541, 60.8847) (50.8498, 60.9002) (48.8424, 60.9131) (46.8319, 60.9234) (44.8187, 60.9308) (42.8034, 60.9354) (40.7866, 60.9371) (38.7685, 60.9357) (36.7493, 60.9313) (34.729, 60.9239) (32.7076, 60.9135) (30.6851, 60.9002) (28.6614, 60.8841) (26.6368, 60.865) (24.6114, 60.843) (22.5853, 60.8181) (20.5589, 60.7901) (18.5322, 60.7592) (16.5056, 60.7253) (14.4789, 60.6883) (12.4525, 60.6483) (10.4264, 60.6052) (8.4007, 60.5591) (6.3754, 60.51) (4.3507, 60.4578) (2.3268, 60.4025) (0.3036, 60.3442) (-1.7185, 60.2827) (-3.7393, 60.2181) (-5.7586, 60.1503) (-7.7762, 60.0792) (-9.7919, 60.0048) (-11.8057, 59.9272) (-13.8177, 59.8464) (-15.8281, 59.7624) (-17.8369, 59.6752) (-19.8438, 59.5848) (-21.8486, 59.4911) (-23.8505, 59.394) (-25.8488, 59.2932) (-27.8429, 59.1888) (-29.8325, 59.0805) (-31.8183, 58.9686) (-33.8013, 58.8532) (-35.7828, 58.7348) (-37.7636, 58.6134) (-39.7435, 58.489) (-41.721, 58.3612) (-43.6928, 58.2294) (-45.6555, 58.0927) (-47.6066, 57.9506) (-49.5462, 57.8031) (-51.4778, 57.651) (-53.4087, 57.4959) (-55.3461, 57.3393) (-57.2945, 57.1824) (-59.2529, 57.0248) (-61.2106, 56.8641) (-63.1498, 56.6964) (-65.0533, 56.5178) (-66.9119, 56.3261) (-68.7305, 56.1225) (-70.538, 55.9134) (-72.3768, 55.7082) (-74.2834, 55.5152) (-76.2727, 55.3377) (-78.3199, 55.1701) (-80.3434, 54.9942) (-82.2424, 54.7874) (-83.9406, 54.5321) (-85.4221, 54.2238) (-86.782, 53.882) (-88.2338, 53.5527) (-90.0202, 53.2939) (-92.3399, 53.1641) (-95.2751, 53.2097) (-98.7005, 53.4518) (-102.322, 53.8868) (-105.7586, 54.4941) (-108.6096, 55.2408) (-110.1447, 55.9181) (-110.7764, 56.453) (-110.9633, 56.8168) (-111, 57) knots 0 0 0 0 0 0 0.00416667 0.00833333 0.0125 0.01666667 0.02083333 0.025 0.02916667 0.03333333 0.0375 0.04166667 0.04583333 0.05 0.05416667 0.05833333 0.0625 0.06666667 0.07083333 0.075 0.07916667 0.08333333 0.0875 0.09166667 0.09583333 0.1 0.10416667 0.10833333 0.1125 0.11666667 0.12083333 0.125 0.12916667 0.13333333 0.1375 0.14166667 0.14583333 0.15 0.15416667 0.15833333 0.1625 0.16666667 0.17083333 0.175 0.17916667 0.18333333 0.1875 0.19166667 0.19583333 0.2 0.20416667 0.20833333 0.2125 0.21666667 0.22083333 0.225 0.22916667 0.23333333 0.2375 0.24166667 0.24583333 0.25 0.25416667 0.25833333 0.2625 0.26666667 0.27083333 0.275 0.27916667 0.28333333 0.2875 0.29166667 0.29583333 0.3 0.30416667 0.30833333 0.3125 0.31666667 0.32083333 0.325 0.32916667 0.33333333 0.3375 0.34166667 0.34583333 0.35 0.35416667 0.35833333 0.3625 0.36666667 0.37083333 0.375 0.37916667 0.38333333 0.3875 0.39166667 0.39583333 0.4 0.40416667 0.40833333 0.4125 0.41666667 0.42083333 0.425 0.42916667 0.43333333 0.4375 0.44166667 0.44583333 0.45 0.45416667 0.45833333 0.4625 0.46666667 0.47083333 0.475 0.47916667 0.48333333 0.4875 0.49166667 0.49583333 0.5 0.50416667 0.50833333 0.5125 0.51666667 0.52083333 0.525 0.52916667 0.53333333 0.5375 0.54166667 0.54583333 0.55 0.55416667 0.55833333 0.5625 0.56666667 0.57083333 0.575 0.57916667 0.58333333 0.5875 0.59166667 0.59583333 0.6 0.60416667 0.60833333 0.6125 0.61666667 0.62083333 0.625 0.62916667 0.63333333 0.6375 0.64166667 0.64583333 0.65 0.65416667 0.65833333 0.6625 0.66666667 0.67083333 0.675 0.67916667 0.68333333 0.6875 0.69166667 0.69583333 0.7 0.70416667 0.70833333 0.7125 0.71666667 0.72083333 0.725 0.72916667 0.73333333 0.7375 0.74166667 0.74583333 0.75 0.75416667 0.75833333 0.7625 0.76666667 0.77083333 0.775 0.77916667 0.78333333 0.7875 0.79166667 0.79583333 0.8 0.80416667 0.80833333 0.8125 0.81666667 0.82083333 0.825 0.82916667 0.83333333 0.8375 0.84166667 0.84583333 0.85 0.85416667 0.85833333 0.8625 0.86666667 0.87083333 0.875 0.87916667 0.88333333 0.8875 0.89166667 0.89583333 0.9 0.90416667 0.90833333 0.9125 0.91666667 0.92083333 0.925 0.92916667 0.93333333 0.9375 0.94166667 0.94583333 0.95 0.95416667 0.95833333 0.9625 0.96666667 0.97083333 0.975 0.97916667 0.98333333 0.9875 0.99166667 0.99583333 1 1 1 1 1 1
  point P0 (-105.4475, 60.7286)
  point P1 (-99.0799, 64.162)
  point P2 (-91.957, 67.2969)
  point P3 (-84.1389, 70.1296)
  point P4 (-75.6853, 72.6568)
  point P5 (-66.6562, 74.875)
  point P6 (-57.1115, 76.7807)
  point P7 (-47.1111, 78.3704)
  point P8 (-36.7148, 79.6406)
  point P9 (-25.9826, 80.588)
  point P10 (-14.9744, 81.2089)
  point P11 (-3.75, 81.5)
  point P12 (7.6306, 81.4578)
  point P13 (19.1076, 81.0787)
  point P14 (30.6211, 80.3594)
  point P15 (42.1111, 79.2963)
  point P16 (53.5178, 77.886)
  point P17 (64.7812, 76.125)
  point P18 (75.8416, 74.0098)
  point P19 (86.6389, 71.537)
  point P20 (97.1133, 68.7031)
  point P21 (107.2049, 65.5046)
  point P22 (116.8537, 61.9381)
  point P23 (126, 58)
  point P24 (117.8078, 58.5935)
  point P25 (109.2541, 59.1233)
  point P26 (100.373, 59.5879)
  point P27 (91.1991, 59.9861)
  point P28 (81.7664, 60.3166)
  point P29 (72.1094, 60.5781)
  point P30 (62.2622, 60.7693)
  point P31 (52.2593, 60.8889)
  point P32 (42.1348, 60.9355)
  point P33 (31.923, 60.908)
  point P34 (21.6583, 60.8049)
  point P35 (11.375, 60.625)
  point P36 (1.1073, 60.367)
  point P37 (-9.1105, 60.0295)
  point P38 (-19.2441, 59.6113)
  point P39 (-29.2593, 59.1111)
  point P40 (-39.1216, 58.5276)
  point P41 (-48.7969, 57.8594)
  point P42 (-58.2508, 57.1053)
  point P43 (-67.4491, 56.2639)
  point P44 (-76.3574, 55.334)
  point P45 (-84.9416, 54.3142)
  point P46 (-93.1672, 53.2033)
extrude "Asymmetric light hood" add sketch "Cantilevered light hood" along normal blind 14 separate body makes body 3 in component "03 Front-Light Hood"
sketch "Hood pins" plane through (0, 0, 0) normal (0, 0, 1) x (1, 0, 0) in component "03 Front-Light Hood"
  circle A0 centre (-50, 75) radius 2
  circle A1 centre (80, 72) radius 2
extrude "Hood pins (1)" add sketch "Hood pins" along normal blind 6 bodies 3 in component "03 Front-Light Hood"
ref_plane "WorkPlane1" through (0, 0, -14.15) normal (0, 0, 1) x (1, 0, 0) in component "04 Opal Diffuser"
sketch "Opal diffuser outline" plane through (0, 0, -14.15) normal (0, 0, 1) x (1, 0, 0) in component "04 Opal Diffuser"
  line L0 (-50.5, 55.05) -> (78.5, 55.05)
  line L1 (80, 56.55) -> (80, 56.75)
  line L2 (78.5, 58.25) -> (-50.5, 58.25)
  line L3 (-52, 56.75) -> (-52, 56.55)
  arc A0 (78.5, 55.05) -> (80, 56.55) centre (78.5, 56.55) ccw
  arc A1 (80, 56.75) -> (78.5, 58.25) centre (78.5, 56.75) ccw
  arc A2 (-50.5, 58.25) -> (-52, 56.75) centre (-50.5, 56.75) ccw
  arc A3 (-52, 56.55) -> (-50.5, 55.05) centre (-50.5, 56.55) ccw
  constraint tangent L0 A0
  constraint tangent L1 A0
  constraint tangent L1 A1
  constraint tangent L2 A1
  constraint tangent L2 A2
  constraint tangent L3 A2
  constraint tangent L3 A3
  constraint tangent L0 A3
extrude "Opal diffuser" add sketch "Opal diffuser outline" along normal blind 5 separate body makes body 4 in component "04 Opal Diffuser"
ref_plane "WorkPlane1" through (0, 0, 3.4) normal (0, 0, 1) x (1, 0, 0) in component "05 Kindle Fit Check (hidden)"
sketch "Kindle body envelope" plane through (0, 0, 3.4) normal (0, 0, 1) x (1, 0, 0) in component "05 Kindle Fit Check (hidden)"
  line L0 (-61.5, -54) -> (94.5, -54)
  line L1 (99.5, -49) -> (99.5, 55)
  line L2 (94.5, 60) -> (-61.5, 60)
  line L3 (-66.5, 55) -> (-66.5, -49)
  arc A0 (94.5, -54) -> (99.5, -49) centre (94.5, -49) ccw
  arc A1 (99.5, 55) -> (94.5, 60) centre (94.5, 55) ccw
  arc A2 (-61.5, 60) -> (-66.5, 55) centre (-61.5, 55) ccw
  arc A3 (-66.5, -49) -> (-61.5, -54) centre (-61.5, -49) ccw
  constraint tangent L0 A0
  constraint tangent L1 A0
  constraint tangent L1 A1
  constraint tangent L2 A1
  constraint tangent L2 A2
  constraint tangent L3 A2
  constraint tangent L3 A3
  constraint tangent L0 A3
extrude "Kindle envelope" add sketch "Kindle body envelope" along normal blind 8.7 separate body makes body 5 in component "05 Kindle Fit Check (hidden)"
sketch "Base plate outline" plane through (0, 0, 0) normal (0, 0, 1) x (1, 0, 0) in component "06 Base Plate (print flat)"
  line L0 (-95, -180) -> (95, -180)
  line L1 (105, -170) -> (105, -110)
  line L2 (95, -100) -> (-95, -100)
  line L3 (-105, -110) -> (-105, -170)
  arc A0 (95, -180) -> (105, -170) centre (95, -170) ccw
  arc A1 (105, -110) -> (95, -100) centre (95, -110) ccw
  arc A2 (-95, -100) -> (-105, -110) centre (-95, -110) ccw
  arc A3 (-105, -170) -> (-95, -180) centre (-95, -170) ccw
  constraint tangent L0 A0
  constraint tangent L1 A0
  constraint tangent L1 A1
  constraint tangent L2 A1
  constraint tangent L2 A2
  constraint tangent L3 A2
  constraint tangent L3 A3
  constraint tangent L0 A3
extrude "Base plate" add sketch "Base plate outline" along normal blind 8 separate body makes body 6 in component "06 Base Plate (print flat)"
ref_plane "WorkPlane1" through (0, 0, 7.8) normal (0, 0, 1) x (1, 0, 0) in component "06 Base Plate (print flat)"
sketch "Rail 1" plane through (0, 0, 7.8) normal (0, 0, 1) x (1, 0, 0) in component "06 Base Plate (print flat)"
  line L0 (-83, -132.3) -> (83, -132.3)
  line L1 (85, -130.3) -> (85, -129.3)
  line L2 (83, -127.3) -> (-83, -127.3)
  line L3 (-85, -129.3) -> (-85, -130.3)
  arc A0 (83, -132.3) -> (85, -130.3) centre (83, -130.3) ccw
  arc A1 (85, -129.3) -> (83, -127.3) centre (83, -129.3) ccw
  arc A2 (-83, -127.3) -> (-85, -129.3) centre (-83, -129.3) ccw
  arc A3 (-85, -130.3) -> (-83, -132.3) centre (-83, -130.3) ccw
  constraint tangent L0 A0
  constraint tangent L1 A0
  constraint tangent L1 A1
  constraint tangent L2 A1
  constraint tangent L2 A2
  constraint tangent L3 A2
  constraint tangent L3 A3
  constraint tangent L0 A3
extrude "Rail 1 (1)" add sketch "Rail 1" along normal blind 8.2 bodies 6 in component "06 Base Plate (print flat)"
sketch "Rail 2" plane through (0, 0, 7.8) normal (0, 0, 1) x (1, 0, 0) in component "06 Base Plate (print flat)"
  line L0 (-83, -152.7) -> (83, -152.7)
  line L1 (85, -150.7) -> (85, -149.7)
  line L2 (83, -147.7) -> (-83, -147.7)
  line L3 (-85, -149.7) -> (-85, -150.7)
  arc A0 (83, -152.7) -> (85, -150.7) centre (83, -150.7) ccw
  arc A1 (85, -149.7) -> (83, -147.7) centre (83, -149.7) ccw
  arc A2 (-83, -147.7) -> (-85, -149.7) centre (-83, -149.7) ccw
  arc A3 (-85, -150.7) -> (-83, -152.7) centre (-83, -150.7) ccw
  constraint tangent L0 A0
  constraint tangent L1 A0
  constraint tangent L1 A1
  constraint tangent L2 A1
  constraint tangent L2 A2
  constraint tangent L3 A2
  constraint tangent L3 A3
  constraint tangent L0 A3
extrude "Rail 2 (1)" add sketch "Rail 2" along normal blind 8.2 bodies 6 in component "06 Base Plate (print flat)"
component "01 Asymmetric Front Shell" placed x (1, 0, 0) y (0, 1, 0) z (0, 0, 1) at (0, 0, 0)
component "02 Rear Cover" placed x (1, 0, 0) y (0, 1, 0) z (0, 0, 1) at (0, 0, 0)
component "03 Front-Light Hood" placed x (1, 0, 0) y (0, 1, 0) z (0, 0, 1) at (0, 0, 0)
component "04 Opal Diffuser" placed x (1, 0, 0) y (0, 1, 0) z (0, 0, 1) at (0, 0, 0)
component "05 Kindle Fit Check (hidden)" placed x (1, 0, 0) y (0, 1, 0) z (0, 0, 1) at (0, 0, 0)
component "06 Base Plate (print flat)" placed x (1, 0, 0) y (0, 1, 0) z (0, 0, 1) at (0, 0, 0)
named bodies: "Asymmetric shell", "Rear cover", "Asymmetric light hood", "Opal diffuser", "Kindle envelope", "Base plate"
